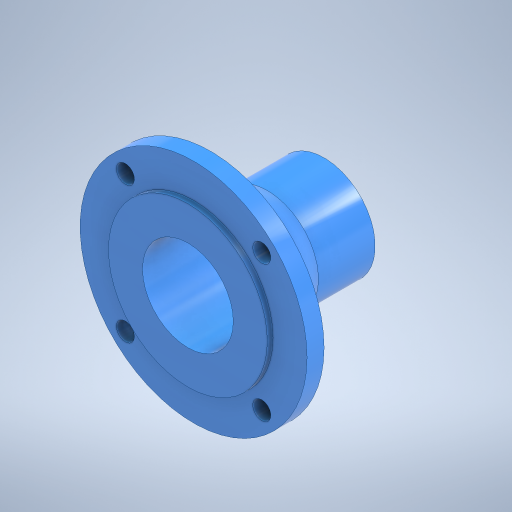
# Autodesk Inventor part: ej_iLogic
Saved by Autodesk Inventor 2023.2 (Build 272271030, 271C)
## iProperties
RuleStatus: InUse
Created: 2023-10-09
Part Number: ej_iLogic
Material: Generic
Document SubType Name: Modeling
Designer: Cris Pat
Density: 1 g/cm^3
Appearance: Cyan
Author: Cris Pat
Autodesk Inventor part; units mm, degrees
ref_plane "YZ Plane" through (0, 0, 0) normal (1, 0, 0) x (0, 1, 0)
ref_plane "XZ Plane" through (0, 0, 0) normal (0, 1, 0) x (-1, 0, 0)
ref_plane "XY Plane" through (0, 0, 0) normal (0, 0, 1) x (1, 0, 0)
sketch "Sketch1" plane through (0, 0, 0) normal (0, 0, 1) x (1, 0, 0)
  circle A0 centre (0, 0) radius 50
  dimension "d_externo" = 100
  constraints: 1 centre point, 1 coincident
  measures "d_externo" diameter of A0
extrude "Extrusion1" add sketch "Sketch1" against normal blind 10
sketch "Sketch2" plane through (0, 0, 0) normal (0, 0, 1) x (1, 0, 0)
  circle A0 centre (0, 0) radius 50 projected
  circle A1 centre (0, 0) radius 35
  dimension "d_resaltado" = 70
  constraints: 1 centre point, 1 coincident
  measures "d_resaltado" diameter of A1
extrude "Extrusion2" cut sketch "Sketch2" against normal blind 2.5
sketch "Sketch3" plane through (0, 0, 0) normal (0, 1, 0) x (-1, 0, 0)
  line L0 (-50, -10) -> (50, -10) construction
  line L1 (35, 0) -> (-35, 0) construction
  line L2 (0, -12) -> (0, 2) projected
  line L3 (0, -10) -> (0, -60)
  line L4 (0, -60) -> (22.5, -60)
  line L5 (22.5, -60) -> (22.5, -35)
  line L6 (22.5, -35) -> (37.5, -10)
  line L7 (37.5, -10) -> (0, -10)
  point P0 (0, 0)
  dimension "d6" = 45
  dimension "d7" = 75
  dimension "d8" = 25
  dimension "d9" = 60
  constraints: 10 end point, 2 collinear, 2 perpendicular
  measures "d6" diameter of L5 L2
  measures "d7" diameter of L6.end L2
  measures "d8" distance from line of L5.end L4
  measures "d9" distance between parallel lines of L1 L4
revolve "Revolution1" add sketch "Sketch3" angle 360 about axis through (0, 0, -10) along (0, 0, 1)
sketch "Sketch4" plane through (0, 0, 0) normal (0, 0, 1) x (1, 0, 0)
  circle A0 centre (0, 0) radius 20
  dimension "d_interior" = 40
  constraints: 1 centre point, 1 coincident
  measures "d_interior" diameter of A0
extrude "Extrusion3" cut sketch "Sketch4" against normal through all
sketch "Sketch5" plane through (0, 0, 0) normal (0, 0, 1) x (1, 0, 0)
  line L0 (0, -70) -> (0, 70) construction
  circle A0 centre (0, 0) radius 42.5 construction
  line L1 (0, 0) -> (30.052, 30.052) construction
  dimension "BCD" = 85
  dimension "ang_a1" = 45
  constraints: 2 coincident, 2 end point, 3 other
  measures "ang_a1" angle of L0 L1
hole "Hole1" at (30.052, 30.052, 0) direction (0, 0, -1) diameter 8 end through all
pattern_circular "Circular Pattern1" count 4 over 360 about axis through (0, 0, -10) along (0, 0, 1) of "Hole1"
body "Solid1"
